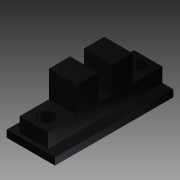
# Autodesk Inventor part: OptoEndStop
Saved by Autodesk Inventor 2014 SP1 (Build 180222100, 222)
## iProperties
Created: 2016-12-01
Part Number: OptoEndStop
Material: Generic
Document SubType Name: Modeling
Designer: danielsikar
Density: 1 g/cm^3
Appearance: Glossy - Black
Author: danielsikar
Autodesk Inventor part; units mm, degrees
ref_plane "YZ Plane" through (0, 0, 0) normal (1, 0, 0) x (0, 1, 0)
ref_plane "XZ Plane" through (0, 0, 0) normal (0, 1, 0) x (-1, 0, 0)
ref_plane "XY Plane" through (0, 0, 0) normal (0, 0, 1) x (1, 0, 0)
sketch "Sketch1" plane through (0, 0, 0) normal (0, 0, 1) x (1, 0, 0)
  line L0 (0, 0) -> (10.2, 0)
  line L1 (10.2, 0) -> (10.2, 25)
  line L2 (10.2, 25) -> (0, 25)
  line L3 (0, 25) -> (0, 0)
  dimension "d0" = 10.2
  dimension "d1" = 25
  constraints: 8 end point, 2 parallel, 1 horizontal, 1 perpendicular
  measures "d0" distance of L2.end L1.end
  measures "d1" distance of L1.end L0.end
extrude "Extrusion1" add sketch "Sketch1" along normal blind 1.5
sketch "Sketch2" plane through (0, 0, 1.5) normal (0, 0, 1) x (1, 0, 0)
  line L0 (10.2, 0) -> (10.2, 25) projected
  line L1 (10.2, 25) -> (0, 25) projected
  line L2 (1.9, 25) -> (7.9, 25)
  line L3 (7.9, 25) -> (7.9, 0.8)
  line L4 (7.9, 0.8) -> (1.9, 0.8)
  line L5 (1.9, 0.8) -> (1.9, 25)
  dimension "d4" = 6
  dimension "d5" = 24.2
  dimension "d6" = 2.3
  dimension "d7" = 0
  constraints: 8 end point, 2 parallel, 1 horizontal, 1 perpendicular
  measures "d4" distance of L3.end L4.end
  measures "d5" distance of L2.end L3.end
  measures "d6" distance between parallel lines of L0 L3
  measures "d7" distance between parallel lines of L1 L2
extrude "Extrusion2" add sketch "Sketch2" along normal blind 3
sketch "Sketch3" plane through (0, 0, 4.5) normal (0, 0, 1) x (1, 0, 0)
  line L0 (1.9, 25) -> (1.9, 0.8) projected
  line L1 (7.9, 0.8) -> (7.9, 25) projected
  line L2 (1.9, 7) -> (7.9, 7)
  line L3 (7.9, 7) -> (7.9, 11.5)
  line L4 (7.9, 11.5) -> (1.9, 11.5)
  line L5 (1.9, 11.5) -> (1.9, 7)
  line L6 (1.9, 14.4) -> (7.9, 14.4)
  line L7 (7.9, 14.4) -> (7.9, 18.7)
  line L8 (7.9, 18.7) -> (1.9, 18.7)
  line L9 (1.9, 18.7) -> (1.9, 14.4)
  line L10 (1.9, 0.8) -> (7.9, 0.8) projected
  point P0 (0, 0)
  dimension "d10" = 4.5
  dimension "d11" = 4.3
  dimension "d12" = 2.9
  dimension "d15" = 6.2
  constraints: 16 end point, 4 parallel, 4 point on line, 2 horizontal, 2 perpendicular
  measures "d10" distance of L3.end L2.end
  measures "d11" distance of L7.end L6.end
  measures "d12" distance between parallel lines of L6 L4
  measures "d15" distance between parallel lines of L2 L10
extrude "Extrusion3" add sketch "Sketch3" along normal blind 5.6 contours L8 L1 L6 L0 | L4 L1 L2 L0
sketch "Sketch4" plane through (0, 0, 4.5) normal (0, 0, 1) x (1, 0, 0)
  line L0 (1.9, 7) -> (1.9, 0.8) projected
  line L1 (1.9, 0.8) -> (7.9, 0.8) projected
  circle A0 centre (4.9, 3.5) radius 1.6
  line L2 (0, 25) -> (0, 0) projected
  dimension "d16" = 3.2
  dimension "d18" = 3
  dimension "d19" = 2.7
  constraints: 1 centre point
  measures "d16" diameter of A0
  measures "d18" distance from line of L0 A0.centre
  measures "d19" distance from line of L1 A0.centre
sketch "Sketch5" plane through (0, 0, 4.5) normal (0, 0, 1) x (1, 0, 0)
  circle A0 centre (4.9, 22.5779) radius 1.6
  circle A1 centre (4.9, 3.4779) radius 1.6
  point P0 (0, 0)
  dimension "d20" = 3.2
  dimension "d21" = 3.2
  dimension "d22" = 19.1
  constraints: 2 centre point
  measures "d20" diameter of A0
  measures "d21" diameter of A1
  measures "d22" distance of A0.centre A1.centre
extrude "Extrusion4" cut sketch "Sketch5" against normal blind 5.6 contours A0
extrude "Extrusion5" cut sketch "Sketch4" against normal blind 5.6
body "Solid1"
